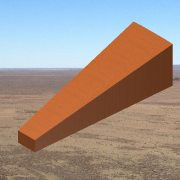
# Autodesk Inventor part: ramp
Saved by Autodesk Inventor 2014 SP1 (Build 180222100, 222)
## iProperties
Created: 2014-05-07
Part Number: ramp
Material: Wood (Cherry)
Document SubType Name: Modeling
Designer: Dave
Density: 0.63 g/cm^3
Appearance: Cherry - Natural Low Gloss
Mass: 109992 g
Surface Area: 27156.6 cm^2
Volume: 174591 cm^3
Author: Dave
Autodesk Inventor part; units mm, degrees
ref_plane "YZ Plane" through (0, 0, 0) normal (1, 0, 0) x (0, 1, 0)
ref_plane "XZ Plane" through (0, 0, 0) normal (0, 1, 0) x (-1, 0, 0)
ref_plane "XY Plane" through (0, 0, 0) normal (0, 0, 1) x (1, 0, 0)
sketch "Sketch1" plane through (0, 0, 0) normal (1, 0, 0) x (0, 1, 0)
  line L0 (0, 0) -> (0, -1524)
  line L1 (0, -1524) -> (431.8, -1524)
  line L2 (0, 0) -> (127, 0)
  line L3 (127, 0) -> (431.8, -1524)
  dimension "d0" = 1524
  dimension "d1" = 431.8
  dimension "d2" = 127
  constraints: 8 end point, 1 parallel, 1 perpendicular, 1 vertical
  measures "d0" distance of L0.start L0.end
  measures "d1" distance of L0.end L1.end
  measures "d2" distance of L0.start L2.end
extrude "Extrusion1" add sketch "Sketch1" along normal blind 203.2
sketch "Sketch2" plane through (203.2, 0, 0) normal (1, 0, 0) x (0, 0, -1)
  line L0 (0, 0) -> (1524, 0) projected
  line L1 (1524, 0) -> (1524, 431.8) projected
  line L2 (1524, 431.8) -> (0, 127) projected
  line L3 (0, 127) -> (0, 0) projected
revolve "Revolution1" add sketch "Sketch2" angle 5 about axis through (203.2, 127, 0) along (0, -1, 0)
sketch "Sketch3" plane through (0, 0, 0) normal (-1, 0, 0) x (0, 0, 1)
  line L0 (0, 0) -> (-1524, 0) projected
  line L1 (0, 127) -> (0, 0) projected
  line L2 (-1524, 431.8) -> (0, 127) projected
  line L3 (-1524, 0) -> (-1524, 431.8) projected
revolve "Revolution2" add sketch "Sketch3" angle 5 about axis through (0, 127, 0) along (0, 1, 0)
body "Solid1"
